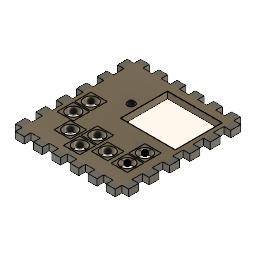
RetroConsoleTop (Autodesk Fusion 360 design; units mm, degrees)
Autodesk Fusion 360 part; units mm, degrees
sketch "Sketch1" plane through (0, 0, 0) normal (0, 0, 1) x (1, 0, 0)
  line L0 (0, 0) -> (74, 0)
  line L1 (74, 0) -> (74, 83)
  line L2 (74, 83) -> (0, 83)
  line L3 (0, 83) -> (0, 0)
  dimension "d1" = 74
  dimension "d2" = 83
  constraint horizontal L0
  constraint vertical L1
  constraint horizontal L2
  constraint vertical L3
  constraint coincident L0.start L3.end
  measures "d1" distance of L0.start L0.end
  measures "d2" distance of L0.start L2.end
extrude "Extrude1" add sketch "Sketch1" along normal blind 5
sketch "Sketch2" plane through (0, 0, 5) normal (0, 0, 1) x (-1, 0, 0)
  line L0 (0, -83) -> (0, 0)
  line L1 (0, 0) -> (-74, 0)
  line L2 (-74, 0) -> (-74, -83)
  line L3 (-74, -83) -> (0, -83)
  line L4 (-30.5, -77.2) -> (-71, -77.2)
  line L5 (-71, -77.2) -> (-71, -42.5)
  line L6 (-71, -42.5) -> (-30.5, -42.5)
  line L7 (-30.5, -42.5) -> (-30.5, -77.2)
  line L8 (-55.8, -22.25) -> (-67.8, -22.25)
  line L9 (-67.8, -22.25) -> (-67.8, -10.25)
  line L10 (-67.8, -10.25) -> (-55.8, -10.25)
  line L11 (-55.8, -10.25) -> (-55.8, -22.25)
  line L12 (-55.8, -35.25) -> (-67.8, -35.25)
  line L13 (-67.8, -35.25) -> (-67.8, -23.25)
  line L14 (-67.8, -23.25) -> (-55.8, -23.25)
  line L15 (-55.8, -23.25) -> (-55.8, -35.25)
  line L16 (-55.8, -29.25) -> (-67.8, -29.25) construction
  line L17 (-61.8, -35.25) -> (-61.8, -23.25) construction
  circle A0 centre (-61.8, -29.25) radius 5
  line L18 (-61.8, -22.25) -> (-61.8, -10.25) construction
  line L19 (-55.8, -16.25) -> (-67.8, -16.25) construction
  circle A1 centre (-61.8, -16.25) radius 5
  line L20 (-25.25, -10.5) -> (-13.25, -10.5)
  line L21 (-13.25, -10.5) -> (-13.25, -22.5)
  line L22 (-13.25, -22.5) -> (-25.25, -22.5)
  line L23 (-25.25, -22.5) -> (-25.25, -10.5)
  circle A2 centre (-19.25, -16.5) radius 5
  line L24 (-38.8, -4) -> (-26.8, -4)
  line L25 (-26.8, -4) -> (-26.8, -16)
  line L26 (-26.8, -16) -> (-38.8, -16)
  line L27 (-38.8, -16) -> (-38.8, -4)
  circle A3 centre (-32.8, -10) radius 5
  line L28 (-38.8, -17) -> (-26.8, -17)
  line L29 (-26.8, -17) -> (-26.8, -29)
  line L30 (-26.8, -29) -> (-38.8, -29)
  line L31 (-38.8, -29) -> (-38.8, -17)
  circle A4 centre (-32.8, -23) radius 5
  line L32 (-53, -10.5) -> (-41, -10.5)
  line L33 (-41, -10.5) -> (-41, -22.5)
  line L34 (-41, -22.5) -> (-53, -22.5)
  line L35 (-53, -22.5) -> (-53, -10.5)
  circle A5 centre (-47, -16.5) radius 5
  line L36 (-14.75, -36.25) -> (-2.75, -36.25)
  line L37 (-2.75, -36.25) -> (-2.75, -48.25)
  line L38 (-2.75, -48.25) -> (-14.75, -48.25)
  line L39 (-14.75, -48.25) -> (-14.75, -36.25)
  circle A6 centre (-8.75, -42.25) radius 5
  line L40 (-14.75, -23.25) -> (-2.75, -23.25)
  line L41 (-2.75, -23.25) -> (-2.75, -35.25)
  line L42 (-2.75, -35.25) -> (-14.75, -35.25)
  line L43 (-14.75, -35.25) -> (-14.75, -23.25)
  circle A7 centre (-8.75, -29.25) radius 5
  circle A8 centre (-25.1, -55.75) radius 2.65
  dimension "d5" = 30.5
  dimension "d6" = 42.5
  dimension "d7" = 34.7
  dimension "d8" = 40.5
  dimension "d11" = 12
  dimension "d14" = 12
  dimension "d15" = 6.2
  dimension "d16" = 10.25
  dimension "d17" = 6.2
  dimension "d19" = 1
  dimension "d20" = 10
  dimension "d21" = 10
  dimension "d22" = 12
  dimension "d23" = 10
  dimension "d24" = 12
  dimension "d25" = 10
  dimension "d26" = 12
  dimension "d27" = 10
  dimension "d28" = 12
  dimension "d29" = 10
  dimension "d32" = 10.5
  dimension "d33" = 6
  dimension "d34" = 6
  dimension "d35" = 4
  dimension "d36" = 6
  dimension "d37" = 6
  dimension "d38" = 21
  dimension "d39" = 17
  dimension "d40" = 6
  dimension "d41" = 6
  dimension "d42" = 35.2
  dimension "d43" = 6
  dimension "d44" = 6
  dimension "d45" = 13.25
  dimension "d46" = 10.5
  dimension "d47" = 12
  dimension "d48" = 10
  dimension "d49" = 6
  dimension "d50" = 6
  dimension "d51" = 12
  dimension "d52" = 10
  dimension "d53" = 6
  dimension "d54" = 6
  dimension "d55" = 2.75
  dimension "d56" = 23.25
  dimension "d57" = 1
  dimension "d58" = 5.3
  dimension "d59" = 27.25
  dimension "d60" = 25.1
  constraint horizontal L4
  constraint vertical L5
  constraint horizontal L6
  constraint vertical L7
  constraint horizontal L8
  constraint vertical L9
  constraint horizontal L10
  constraint vertical L11
  constraint equal L9 L10
  constraint horizontal L12
  constraint vertical L13
  constraint horizontal L14
  constraint vertical L15
  constraint equal L13 L14
  constraint midpoint L15 L16.start
  constraint midpoint L13 L16.end
  constraint midpoint L12 L17.start
  constraint midpoint L14 L17.end
  constraint midpoint L16 A0.centre
  constraint midpoint L8 L18.start
  constraint midpoint L10 L18.end
  constraint midpoint L11 L19.start
  constraint midpoint L9 L19.end
  constraint midpoint L19 A1.centre
  constraint horizontal L22
  constraint vertical L23
  constraint horizontal L20
  constraint vertical L21
  constraint equal L20 L23
  constraint horizontal L26
  constraint vertical L27
  constraint horizontal L24
  constraint vertical L25
  constraint equal L24 L27
  constraint horizontal L30
  constraint vertical L31
  constraint horizontal L28
  constraint vertical L29
  constraint equal L28 L31
  constraint horizontal L34
  constraint vertical L35
  constraint horizontal L32
  constraint vertical L33
  constraint equal L32 L35
  constraint collinear L25 L29
  constraint horizontal L38
  constraint vertical L39
  constraint horizontal L36
  constraint vertical L37
  constraint equal L36 L39
  constraint horizontal L42
  constraint vertical L43
  constraint horizontal L40
  constraint vertical L41
  constraint equal L40 L43
  constraint collinear L37 L41
  measures "d5" distance of L0 L6.end
  measures "d6" distance of L1 L5.end
  measures "d7" distance of L4.end L5.end
  measures "d8" distance of L5.end L6.end
  measures "d11" distance of L9.end L8.end
  measures "d14" distance of L13.end L12.end
  measures "d15" distance of L2 L9
  measures "d16" distance of L1 L10
  measures "d17" distance of L2 L13
  measures "d19" distance of L8.start L14.end
  measures "d20" diameter of A0
  measures "d21" diameter of A1
  measures "d22" distance of L22.end L20.start
  measures "d23" diameter of A2
  measures "d24" distance of L26.end L24.start
  measures "d25" diameter of A3
  measures "d26" distance of L30.end L28.start
  measures "d27" diameter of A4
  measures "d28" distance of L34.end L32.start
  measures "d29" diameter of A5
  measures "d32" distance of L1 L32.end
  measures "d33" distance of A5.centre L33
  measures "d34" distance of A5.centre L34
  measures "d35" distance of L1 L24
  measures "d36" distance of A3.centre L25
  measures "d37" distance of A3.centre L26
  measures "d38" distance of L2 L35
  measures "d39" distance of L1 L28
  measures "d40" distance of A4.centre L29
  measures "d41" distance of A4.centre L30
  measures "d42" distance of L2 L27
  measures "d43" distance of A2.centre L21
  measures "d44" distance of A2.centre L22
  measures "d45" distance of L0 L21
  measures "d46" distance of L1 L20
  measures "d47" distance of L36.start L38.end
  measures "d48" diameter of A6
  measures "d49" distance of A6.centre L37
  measures "d50" distance of A6.centre L38
  measures "d51" distance of L40.start L42.end
  measures "d52" diameter of A7
  measures "d53" distance of A7.centre L41
  measures "d54" distance of A7.centre L42
  measures "d55" distance of L0 L37
  measures "d56" distance of L1 L40
  measures "d57" distance of L36 L42
  measures "d58" diameter of A8
  measures "d59" distance of L3 A8.centre
  measures "d60" distance of L0 A8.centre
extrude "Extrude3" cut sketch "Sketch2" against normal blind 5 contours A8
extrude "Extrude2" cut sketch "Sketch2" against normal blind 5 contours L4 L5 L6 L7 | A0 | A1 | A2 | A3 | A4 | A5 | A6 | A7
sketch "Sketch3" plane through (74, 0, 0) normal (1, 0, 0) x (0, 1, 0)
  line L0 (0, 0) -> (83, 0)
  line L1 (83, 0) -> (83, 5)
  line L2 (83, 5) -> (0, 5)
  line L3 (0, 5) -> (0, 0)
  line L4 (0, 5) -> (7.4455, 5)
  line L5 (7.4455, 5) -> (7.4455, 0)
  line L6 (7.4455, 0) -> (0, 0)
  line L7 (0, 0) -> (0, 5)
  line L8 (15.1109, 0) -> (15.1109, 5)
  line L9 (15.1109, 5) -> (22.5564, 5)
  line L10 (22.5564, 5) -> (22.5564, 0)
  line L11 (22.5564, 0) -> (15.1109, 0)
  line L12 (30.2218, 0) -> (30.2218, 5)
  line L13 (30.2218, 5) -> (37.6673, 5)
  line L14 (37.6673, 5) -> (37.6673, 0)
  line L15 (37.6673, 0) -> (30.2218, 0)
  line L16 (45.3327, 0) -> (45.3327, 5)
  line L17 (45.3327, 5) -> (52.7782, 5)
  line L18 (52.7782, 5) -> (52.7782, 0)
  line L19 (52.7782, 0) -> (45.3327, 0)
  line L20 (60.4436, 0) -> (60.4436, 5)
  line L21 (60.4436, 5) -> (67.8891, 5)
  line L22 (67.8891, 5) -> (67.8891, 0)
  line L23 (67.8891, 0) -> (60.4436, 0)
  line L24 (75.5545, 0) -> (75.5545, 5)
  line L25 (75.5545, 5) -> (83, 5)
  line L26 (83, 5) -> (83, 0)
  line L27 (83, 0) -> (75.5545, 0)
  dimension "d70" = 7.4455
  dimension "d74" = 75.5545
  dimension "d75" = 0
  constraint horizontal L4
  constraint vertical L5
  constraint horizontal L6
  constraint vertical L7
  constraint coincident L2 L3.start
  constraint coincident L0.start L3.end
  measures "d70" distance of L2.end L4.end
extrude "Extrude4" add sketch "Sketch3" along normal blind 5 contours L0 L2 L3 L4 L5 L6 L7 | L0 L2 L8 L9 L10 L11 | L0 L2 L12 L13 L14 L15 | L0 L2 L16 L17 L18 L19 | L0 L2 L20 L21 L22 L23 | L0 L1 L2 L24 L25 L26 L27
sketch "Sketch4" plane through (0, 0, 0) normal (-1, 0, 0) x (0, -1, 0)
  line L0 (-83, 0) -> (0, 0)
  line L1 (0, 0) -> (0, 5)
  line L2 (0, 5) -> (-83, 5)
  line L3 (-83, 5) -> (-83, 0)
  line L4 (-83, 5) -> (-75.5545, 5)
  line L5 (-75.5545, 5) -> (-75.5545, 0)
  line L6 (-75.5545, 0) -> (-83, 0)
  line L7 (-83, 0) -> (-83, 5)
  line L8 (-67.8891, 0) -> (-67.8891, 5)
  line L9 (-67.8891, 5) -> (-60.4436, 5)
  line L10 (-60.4436, 5) -> (-60.4436, 0)
  line L11 (-60.4436, 0) -> (-67.8891, 0)
  line L12 (-52.7782, 0) -> (-52.7782, 5)
  line L13 (-52.7782, 5) -> (-45.3327, 5)
  line L14 (-45.3327, 5) -> (-45.3327, 0)
  line L15 (-45.3327, 0) -> (-52.7782, 0)
  line L16 (-37.6673, 0) -> (-37.6673, 5)
  line L17 (-37.6673, 5) -> (-30.2218, 5)
  line L18 (-30.2218, 5) -> (-30.2218, 0)
  line L19 (-30.2218, 0) -> (-37.6673, 0)
  line L20 (-22.5564, 0) -> (-22.5564, 5)
  line L21 (-22.5564, 5) -> (-15.1109, 5)
  line L22 (-15.1109, 5) -> (-15.1109, 0)
  line L23 (-15.1109, 0) -> (-22.5564, 0)
  line L24 (-7.4455, 0) -> (-7.4455, 5)
  line L25 (-7.4455, 5) -> (0, 5)
  line L26 (0, 5) -> (0, 0)
  line L27 (0, 0) -> (-7.4455, 0)
  dimension "d78" = 7.4455
  dimension "d81" = 75.5545
  dimension "d82" = 0
  constraint horizontal L4
  constraint vertical L5
  constraint horizontal L6
  constraint vertical L7
  constraint coincident L0 L5.end
  constraint coincident L2 L3.start
  constraint coincident L0.start L3.end
  measures "d78" distance of L2.end L4.end
extrude "Extrude5" add sketch "Sketch4" along normal blind 5 contours L0 L2 L3 L4 L5 L6 L7 | L0 L2 L8 L9 L10 L11 | L0 L2 L12 L13 L14 L15 | L0 L2 L16 L17 L18 L19 | L0 L2 L20 L21 L22 L23 | L0 L1 L2 L24 L25 L26 L27
sketch "Sketch5" plane through (0, 0, 0) normal (0, -1, 0) x (1, 0, 0)
  line L0 (-5, 0) -> (79, 0)
  line L1 (79, 0) -> (79, 5)
  line L2 (79, 5) -> (-5, 5)
  line L3 (-5, 5) -> (-5, 0)
  line L4 (0, 5) -> (6.6273, 5)
  line L5 (6.6273, 5) -> (6.6273, 0)
  line L6 (6.6273, 0) -> (0, 0)
  line L7 (0, 0) -> (0, 5)
  line L8 (13.4745, 0) -> (13.4745, 5)
  line L9 (13.4745, 5) -> (20.1018, 5)
  line L10 (20.1018, 5) -> (20.1018, 0)
  line L11 (20.1018, 0) -> (13.4745, 0)
  line L12 (26.9491, 0) -> (26.9491, 5)
  line L13 (26.9491, 5) -> (33.5764, 5)
  line L14 (33.5764, 5) -> (33.5764, 0)
  line L15 (33.5764, 0) -> (26.9491, 0)
  line L16 (40.4236, 0) -> (40.4236, 5)
  line L17 (40.4236, 5) -> (47.0509, 5)
  line L18 (47.0509, 5) -> (47.0509, 0)
  line L19 (47.0509, 0) -> (40.4236, 0)
  line L20 (53.8982, 0) -> (53.8982, 5)
  line L21 (53.8982, 5) -> (60.5255, 5)
  line L22 (60.5255, 5) -> (60.5255, 0)
  line L23 (60.5255, 0) -> (53.8982, 0)
  line L24 (67.3727, 0) -> (67.3727, 5)
  line L25 (67.3727, 5) -> (74, 5)
  line L26 (74, 5) -> (74, 0)
  line L27 (74, 0) -> (67.3727, 0)
  point P0 (0, 5)
  dimension "d85" = 6.6273
  dimension "d88" = 67.3727
  dimension "d89" = 0
  constraint horizontal L4
  constraint vertical L5
  constraint horizontal L6
  constraint vertical L7
  constraint coincident L0 L5.end
  constraint coincident P0 L4.start
  measures "d85" distance of P0 L4.end
extrude "Extrude6" add sketch "Sketch5" along normal blind 5 contours L0 L2 L4 L5 L6 L7 | L0 L2 L8 L9 L10 L11 | L0 L2 L12 L13 L14 L15 | L0 L2 L16 L17 L18 L19 | L0 L2 L20 L21 L22 L23 | L0 L2 L24 L25 L26 L27
sketch "Sketch6" plane through (0, 83, 0) normal (0, 1, 0) x (-1, 0, 0)
  line L0 (-79, 0) -> (5, 0)
  line L1 (5, 0) -> (5, 5)
  line L2 (5, 5) -> (-79, 5)
  line L3 (-79, 5) -> (-79, 0)
  line L4 (-74, 5) -> (-67.3727, 5)
  line L5 (-67.3727, 5) -> (-67.3727, 0)
  line L6 (-67.3727, 0) -> (-74, 0)
  line L7 (-74, 0) -> (-74, 5)
  line L8 (-60.5255, 0) -> (-60.5255, 5)
  line L9 (-60.5255, 5) -> (-53.8982, 5)
  line L10 (-53.8982, 5) -> (-53.8982, 0)
  line L11 (-53.8982, 0) -> (-60.5255, 0)
  line L12 (-47.0509, 0) -> (-47.0509, 5)
  line L13 (-47.0509, 5) -> (-40.4236, 5)
  line L14 (-40.4236, 5) -> (-40.4236, 0)
  line L15 (-40.4236, 0) -> (-47.0509, 0)
  line L16 (-33.5764, 0) -> (-33.5764, 5)
  line L17 (-33.5764, 5) -> (-26.9491, 5)
  line L18 (-26.9491, 5) -> (-26.9491, 0)
  line L19 (-26.9491, 0) -> (-33.5764, 0)
  line L20 (-20.1018, 0) -> (-20.1018, 5)
  line L21 (-20.1018, 5) -> (-13.4745, 5)
  line L22 (-13.4745, 5) -> (-13.4745, 0)
  line L23 (-13.4745, 0) -> (-20.1018, 0)
  line L24 (-6.6273, 0) -> (-6.6273, 5)
  line L25 (-6.6273, 5) -> (0, 5)
  line L26 (0, 5) -> (0, 0)
  line L27 (0, 0) -> (-6.6273, 0)
  point P0 (-74, 5)
  point P1 (-67.3727, 0)
  dimension "d94" = 67.3727
  dimension "d95" = 0
  constraint horizontal L4
  constraint vertical L5
  constraint horizontal L6
  constraint vertical L7
  constraint coincident P1 L5.end
  constraint coincident P0 L4.start
extrude "Extrude7" add sketch "Sketch6" along normal blind 5 contours L0 L2 L4 L5 L6 L7 | L0 L2 L8 L9 L10 L11 | L0 L2 L12 L13 L14 L15 | L0 L2 L16 L17 L18 L19 | L0 L2 L20 L21 L22 L23 | L0 L2 L24 L25 L26 L27
equation "pikkus = 83 mm"
equation "laius = 74 mm"
equation "paksus = 5 mm"
equation "pikkus_tapp = pikkus / 11 - 0.1 mm"
equation "laius_tapp = laius / 11 - 0.1 mm"
equation "d70 = pikkus_tapp"
equation "d74 = pikkus - pikkus_tapp"
equation "d76 = paksus"
equation "d78 = pikkus_tapp"
equation "d81 = pikkus - pikkus_tapp"
equation "d83 = paksus"
equation "d85 = laius_tapp"
equation "d88 = laius - laius_tapp"
equation "d90 = paksus"
equation "d94 = laius - laius_tapp"
equation "d96 = paksus"
